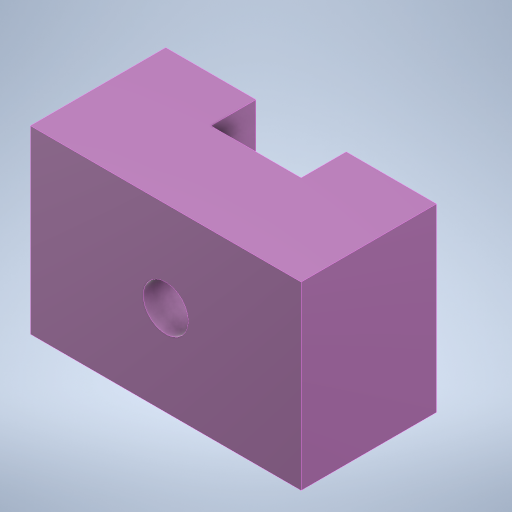
# Autodesk Inventor part: trzymaczka
Saved by Autodesk Inventor 2024 (Build 280153000, 153)
## iProperties
Created: 2024-08-23
Part Number: trzymaczka
Material: Generic
Document SubType Name: Modeling
Designer: domko
Density: 1 g/cm^3
Appearance: Smooth - Purple
Author: domko
Autodesk Inventor part; units mm, degrees
ref_plane "YZ Plane" through (0, 0, 0) normal (1, 0, 0) x (0, 1, 0)
ref_plane "XZ Plane" through (0, 0, 0) normal (0, 1, 0) x (-1, 0, 0)
ref_plane "XY Plane" through (0, 0, 0) normal (0, 0, 1) x (1, 0, 0)
sketch "Sketch1" plane through (0, 0, 0) normal (0, 0, 1) x (1, 0, 0)
  line L0 (-30, 20) -> (30, 20)
  line L1 (30, 20) -> (30, -20)
  line L2 (30, -20) -> (-30, -20)
  line L3 (-30, -20) -> (-30, 20)
  point P0 (0, 0)
  dimension "d0" = 60
  dimension "d1" = 30
  dimension "d2" = 40
  dimension "d3" = 20
  constraints: 8 end point, 2 parallel, 1 horizontal, 1 perpendicular
  measures "d0" distance between parallel lines of L1 L3
  measures "d1" distance from line of L3 point (0, 0)
  measures "d2" distance between parallel lines of L0 L2
  measures "d3" distance from line of point (0, 0) L0
extrude "Extrusion1" add sketch "Sketch1" along normal blind 30
sketch "Sketch3" plane through (-30, 20, 0) normal (0, 1, 0) x (1, 0, 0)
  line L0 (0, 0) -> (60, 0) projected
  line L1 (20, 0) -> (20, -10)
  line L2 (20, -10) -> (40, -10)
  line L3 (40, -10) -> (40, 0)
  line L4 (20, 0) -> (40, 0)
  point P0 (30, 0)
  point P1 (30, 0)
  dimension "d9" = 20
  dimension "d10" = 10
  dimension "d11" = 10
  constraints: 8 end point, 2 perpendicular, 2 point on line, 1 collinear, 1 midpoint, 1 vertical
  measures "d9" distance of L1.end L2.end
  measures "d10" distance from line of L1 point (30, 0)
  measures "d11" distance between parallel lines of L0 L2
extrude "Extrusion3" cut sketch "Sketch3" against normal through all
sketch "Sketch5" plane through (10, 20, 10) normal (0, 0, -1) x (-1, 0, 0)
  line L0 (12.5, -22.5) -> (7.5, -22.5)
  line L1 (7.5, -22.5) -> (7.5, -17.5)
  line L2 (7.5, -17.5) -> (12.5, -17.5)
  line L3 (12.5, -17.5) -> (12.5, -22.5)
  point P0 (10, -20)
  point P1 (7.5, -20)
  dimension "d17" = 2.5
  dimension "d18" = 5
  dimension "d19" = 5
  dimension "d20" = 2.5
  constraints: 8 end point, 2 parallel, 1 horizontal, 1 midpoint, 1 perpendicular
  measures "d17" distance of point (7.5, -20) point (10, -20)
  measures "d18" distance of L0.start L0.end
  measures "d19" distance of L0.end L1.end
  measures "d20" distance from line of L0 point (10, -20)
extrude "Extrusion5" add sketch "Sketch5" along normal blind 20
sketch "Sketch6" plane through (0, 0, 30) normal (0, 0, 1) x (1, 0, 0)
  circle A0 centre (0, 0) radius 5
  dimension "d23" = 10
  constraints: 1 centre point, 1 coincident
  measures "d23" diameter of A0
extrude "Extrusion6" cut sketch "Sketch6" against normal blind 10
body "Solid1"
